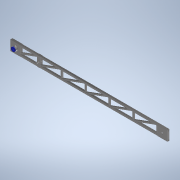
# Autodesk Inventor part: ms truss - 2
Saved by Autodesk Inventor 2020 (Build 240168000, 168)
## iProperties
Created: 2020-07-25
Part Number: ms truss - 2
Material: Steel, Mild
Document SubType Name: Modeling
Designer: Vikki
Mass: 14529.5 g
Surface Area: 14203.7 cm^2
Volume: 1850.9 cm^3
Density: 7.85 g/cm^3
Appearance: Semi-Polished
Author: Vikki
Autodesk Inventor part; units mm, degrees
ref_plane "YZ Plane" through (0, 0, 0) normal (1, 0, 0) x (0, 1, 0)
ref_plane "XZ Plane" through (0, 0, 0) normal (0, 1, 0) x (-1, 0, 0)
ref_plane "XY Plane" through (0, 0, 0) normal (0, 0, 1) x (1, 0, 0)
sketch "Sketch1" plane through (0, 0, 0) normal (1, 0, 0) x (0, 1, 0)
  line L0 (-12.7, 12.7) -> (12.7, 12.7)
  line L1 (12.7, 12.7) -> (12.7, -12.7)
  line L2 (12.7, -12.7) -> (-12.7, -12.7)
  line L3 (-12.7, -12.7) -> (-12.7, 12.7)
  line L4 (-12.7, 12.7) -> (12.7, -12.7) construction
  line L5 (12.7, 12.7) -> (-12.7, -12.7) construction
  line L6 (11.1, 11.1) -> (-11.1, 11.1)
  line L7 (-11.1, 11.1) -> (-11.1, -11.1)
  line L8 (-11.1, -11.1) -> (11.1, -11.1)
  line L9 (11.1, -11.1) -> (11.1, 11.1)
  line L10 (114.3, -11.1) -> (136.5, -11.1)
  line L11 (136.5, -11.1) -> (136.5, 11.1)
  line L12 (136.5, 11.1) -> (114.3, 11.1)
  line L13 (114.3, 11.1) -> (114.3, -11.1)
  line L14 (114.3, -11.1) -> (136.5, 11.1) construction
  line L15 (136.5, -11.1) -> (114.3, 11.1) construction
  line L16 (112.7, -12.7) -> (138.1, -12.7)
  line L17 (138.1, -12.7) -> (138.1, 12.7)
  line L18 (138.1, 12.7) -> (112.7, 12.7)
  line L19 (112.7, 12.7) -> (112.7, -12.7)
  line L20 (112.7, -12.7) -> (138.1, 12.7) construction
  line L21 (138.1, -12.7) -> (112.7, 12.7) construction
  point P0 (0, 0)
  point P1 (125.4, 0)
  point P2 (0, 0)
  point P3 (125.4, 0)
  dimension "d0" = 25.4
  dimension "d1" = 25.4
  dimension "d2" = 1.6
  dimension "d5" = 125.4
  constraints: 44 end point, 8 midpoint, 8 parallel, 4 equal length, 4 perpendicular, 3 horizontal, 1 horizontal alignment, 3 other
  measures "d0" distance of L1.end L2.end
  measures "d1" distance of L0.end L1.end
  measures "d2" distance between parallel lines of L0 L6
  measures "d5" distance of point (0, 0) point (125.4, 0)
extrude "Extrusion1" add sketch "Sketch1" along normal blind 2000
sketch "Sketch2" plane through (0, 12.7, 12.7) normal (0, 1, 0) x (1, 0, 0)
  line L0 (0, 25.4) -> (2000, 25.4) projected
  line L1 (0, 0) -> (25.4, 0)
  line L2 (25.4, 0) -> (25.4, 25.4)
  line L3 (25.4, 25.4) -> (0, 25.4)
  line L4 (0, 25.4) -> (0, 0)
  line L5 (2, 2) -> (23.4, 2)
  line L6 (23.4, 2) -> (23.4, 23.4)
  line L7 (23.4, 23.4) -> (2, 23.4)
  line L8 (2, 23.4) -> (2, 2)
  line L9 (2000, 0) -> (1974.6, 0)
  line L10 (1974.6, 0) -> (1974.6, 25.4)
  line L11 (1974.6, 25.4) -> (2000, 25.4)
  line L12 (2000, 25.4) -> (2000, 0)
  line L13 (1976.2, 1.6) -> (1998.4, 1.6)
  line L14 (1998.4, 1.6) -> (1998.4, 23.8)
  line L15 (1998.4, 23.8) -> (1976.2, 23.8)
  line L16 (1976.2, 23.8) -> (1976.2, 1.6)
  point P0 (0, 12.7)
  dimension "d6" = 25.4
  dimension "d7" = 2
  dimension "d8" = 25.4
  dimension "d9" = 1.6
  constraints: 32 end point, 8 parallel, 4 perpendicular, 2 horizontal, 2 point on line, 6 other
  measures "d6" distance of L1.start L1.end
  measures "d7" distance between parallel lines of L4 L8
  measures "d8" distance of L9.start L9.end
  measures "d9" distance between parallel lines of L13 L9
extrude "Extrusion2" add sketch "Sketch2" along normal up to surface (100 mm away)
sketch "Sketch3" plane through (25.4, 12.7, -12.7) normal (0, 1, 0) x (1, 0, 0)
  line L0 (90.2984, -21.425) -> (34.6, -21.425)
  line L1 (34.6, -21.425) -> (34.6, -2.375)
  line L2 (34.6, -2.375) -> (90.2984, -2.375)
  line L3 (90.2984, -2.375) -> (90.2984, -21.425)
  line L4 (-25.4, -23.8) -> (1974.6, -23.8) projected
  line L5 (-25.4, -23.8) -> (-25.4, -1.6) projected
  line L6 (89.0984, -20.225) -> (35.8, -20.225)
  line L7 (35.8, -20.225) -> (35.8, -3.575)
  line L8 (35.8, -3.575) -> (89.0984, -3.575)
  line L9 (89.0984, -3.575) -> (89.0984, -20.225)
  point P0 (-25.4, -12.7)
  point P1 (71.2484, -11.9)
  dimension "d12" = 19.05
  dimension "d13" = 55.6984
  dimension "d14" = 2.375
  dimension "d15" = 60
  dimension "d16" = 1.2
  dimension "d17" = 19.05
  dimension "d18" = 9.525
  constraints: 16 end point, 4 parallel, 2 perpendicular, 1 horizontal, 3 other
  measures "d12" distance of L0.end L1.end
  measures "d13" distance of L0.start L0.end
  measures "d14" distance between parallel lines of L0 L4
  measures "d15" distance between parallel lines of L1 L5
  measures "d16" distance between parallel lines of L3 L9
  measures "d17" distance from line of L3 point (71.248, -11.9)
  measures "d18" distance from line of L0 point (71.248, -11.9)
sketch "Sketch5" plane through (25.4, 112.7, 12.7) normal (0, -1, 0) x (1, 0, 0)
  point P0 (-25.4, -12.7)
  point P1 (71.2484, -13.5)
  point P2 (345.9961, -13.5)
  dimension "d19" = 274.7477
  constraints: 1 horizontal alignment
  measures "d19" distance of point (345.996, -13.5) point (71.248, -13.5)
sketch3d "3D Sketch1"
  line L0 (96.6484, 12.7, -0.8) -> (371.3961, 112.7, -0.8)
sweep "Sweep1" add profiles "Sketch3" path "3D Sketch1"
sketch "Sketch13" plane through (2000, -12.7, 12.7) normal (0, 0, 1) x (1, 0, 0)
  line L0 (0, 0) -> (-150, 0)
  line L1 (-150, 0) -> (-150, 150.8)
  line L2 (-150, 150.8) -> (0, 150.8)
  line L3 (0, 150.8) -> (0, 0)
  line L4 (-2000, 150.8) -> (0, 150.8) projected
  point P0 (-2000, 12.7)
  dimension "d60" = 150
  dimension "d133" = 0
  constraints: 8 end point, 2 parallel, 1 horizontal, 1 perpendicular
  measures "d60" distance of L1.end L2.end
  measures "d133" distance between parallel lines of L2 L4
sketch "Sketch17" plane through (25.4, 112.7, 12.7) normal (0, -1, 0) x (1, 0, 0)
  line L0 (370.0461, -3.975) -> (389.0961, -3.975)
  line L1 (389.0961, -3.975) -> (389.0961, -23.025)
  line L2 (389.0961, -23.025) -> (370.0461, -23.025)
  line L3 (370.0461, -23.025) -> (370.0461, -3.975)
  line L4 (309.3477, -3.975) -> (365.0461, -3.975) projected
  line L5 (365.0461, -23.025) -> (309.3477, -23.025) projected
  line L6 (365.0461, -3.975) -> (365.0461, -23.025) projected
  line L7 (371.0711, -22) -> (388.0711, -22)
  line L8 (388.0711, -22) -> (388.0711, -5)
  line L9 (388.0711, -5) -> (371.0711, -5)
  line L10 (371.0711, -5) -> (371.0711, -22)
  point P0 (-25.4, -12.7)
  dimension "d73" = 0
  dimension "d74" = 0
  dimension "d75" = 5
  dimension "d76" = 1.025
  constraints: 16 end point, 4 parallel, 3 perpendicular, 1 horizontal, 3 other
  measures "d73" distance between parallel lines of L0 L4
  measures "d74" distance between parallel lines of L5 L2
  measures "d75" distance between parallel lines of L6 L3
  measures "d76" distance between parallel lines of L2 L7
extrude "Extrusion14" add sketch "Sketch17" along normal up to surface (100 mm away)
pattern_linear "Rectangular Pattern3" count 5 spacing 357 along (1, 0, 0) of "Sweep1", "Extrusion14"
sketch "Sketch18" plane through (0, 0, 0) normal (-1, 0, 0) x (0, 0, 1)
  line L0 (-11.1, 136.5) -> (-11.1, 114.3) projected
  line L1 (11.1, 136.5) -> (-11.1, 136.5) projected
  line L2 (11.1, 114.3) -> (11.1, 136.5) projected
  line L3 (-11.1, 114.3) -> (11.1, 114.3) projected
  line L4 (12.7, 138.1) -> (12.7, -12.7) projected
  line L5 (-12.7, 138.1) -> (12.7, 138.1) projected
  line L6 (-12.7, -12.7) -> (-12.7, 138.1) projected
  line L7 (12.7, -12.7) -> (-12.7, -12.7) projected
  line L8 (-11.1, -11.1) -> (11.1, -11.1) projected
  line L9 (-11.1, 11.1) -> (-11.1, -11.1) projected
  line L10 (11.1, 11.1) -> (-11.1, 11.1) projected
  line L11 (11.1, -11.1) -> (11.1, 11.1) projected
  line L12 (-12.7, -12.7) -> (-12.7, 138.1) projected
  line L13 (-12.7, 112.7) -> (12.7, 112.7)
  line L14 (12.7, 138.1) -> (12.7, -12.7) projected
  line L15 (-12.7, 12.7) -> (12.7, 12.7)
  point P0 (0, 0)
  dimension "d82" = 1.6
  dimension "d83" = 1.6
  constraints: 4 end point, 4 point on line, 2 perpendicular
  measures "d82" distance between parallel lines of L13 L3
  measures "d83" distance between parallel lines of L10 L15
extrude "Extrusion15" add sketch "Sketch18" along normal blind 350 contours L4 L13 L6 L5 | L4 L7 L6 L15
sketch "Sketch20" plane through (25.4, 12.7, -12.7) normal (0, 0, -1) x (-1, 0, 0)
  line L0 (0, 0) -> (0, 100) projected
  line L1 (25.4, 0) -> (25.4, 100) projected
  line L2 (0, 100) -> (25.4, 100)
  line L3 (25.4, 100) -> (25.4, 0)
  line L4 (25.4, 0) -> (0, 0)
  line L5 (0, 0) -> (0, 100)
  point P0 (25.4, -12.7)
  point P1 (25.4, 100)
  constraints: 8 end point, 2 parallel, 1 horizontal, 1 perpendicular
extrude "Extrusion16" cut sketch "Sketch20" against normal blind 350
ref_plane "Work Plane5" through (1850, -12.7, -12.7) normal (0, 0, -1) x (-1, 0, 0)
sketch "Sketch22" plane through (1850, -12.7, -12.7) normal (0, 0, -1) x (-1, 0, 0)
  circle A0 centre (2125, 75.4) radius 15 projected
  line L0 (2200, 150.8) -> (0, 150.8) projected
  line L1 (2200, 1.6) -> (2050, 1.6)
  line L2 (2050, 1.6) -> (2050, 150.8)
  line L3 (2050, 150.8) -> (2200, 150.8)
  line L4 (2200, 150.8) -> (2200, 1.6)
  point P0 (1850, 12.7)
  point P1 (0, 150.8)
  dimension "d96" = 150
  constraints: 8 end point, 2 parallel, 1 horizontal, 1 perpendicular, 1 point on line
  measures "d96" distance of L1.start L1.end
extrude "Extrusion18" add sketch "Sketch22" along normal blind 4
sketch "Sketch23" plane through (-350, -12.7, 12.7) normal (0, 0, 1) x (1, 0, 0)
  line L0 (150, 1.6) -> (0, 1.6) projected
  line L1 (0, 1.6) -> (0, 150.8) projected
  line L2 (0, 150.8) -> (150, 150.8) projected
  line L3 (150, 150.8) -> (150, 1.6) projected
  circle A0 centre (75, 75.4) radius 15 projected
  point P0 (350, 12.7)
extrude "Extrusion19" add sketch "Sketch23" along normal blind 4
sketch "Sketch24" plane through (-350, -12.7, 16.7) normal (0, 0, 1) x (1, 0, 0)
  line L0 (150, 150.8) -> (0, 150.8) projected
  line L1 (0, 150.8) -> (0, 1.6) projected
  line L2 (0, 1.6) -> (150, 1.6) projected
  line L3 (150, 1.6) -> (150, 150.8) projected
  circle A0 centre (75, 75.4) radius 15 projected
  circle A1 centre (75, 75.4) radius 35
  circle A2 centre (75, 75.4) radius 31
  point P0 (350, 12.7)
  dimension "d101" = 70
  dimension "d104" = 62
  constraints: 2 centre point, 2 coincident
  measures "d101" diameter of A1
  measures "d104" diameter of A2
extrude "Extrusion20" add sketch "Sketch24" along normal blind 25 contours A1
sketch "Sketch26" plane through (1850, -12.7, -16.7) normal (0, 0, -1) x (-1, 0, 0)
  circle A0 centre (2125, 75.4) radius 35 projected
  circle A1 centre (2125, 75.4) radius 31 projected
  point P0 (1850, 12.7)
extrude "Extrusion21" add sketch "Sketch26" along normal blind 25
fillet "Fillet1" radius 8 1 edges at (-310, 62.7, 16.7)
fillet "Fillet3" radius 5 2 edges at (-200, 125.4, 12.7) (-200, 0.8, 12.7)
sketch "Sketch28" plane through (-350, -12.7, 12.7) normal (0, 0, 1) x (1, 0, 0)
  circle A0 centre (425, 75.4) radius 12.5
  circle A1 centre (75, 75.4) radius 15 projected
  point P0 (350, 12.7)
  dimension "d110" = 350
  dimension "d111" = 25
  dimension "d126" = 0
  constraints: 1 centre point
  measures "d110" distance of A0.centre A1.centre
  measures "d111" diameter of A0
  measures "d126" vertical distance of A1.centre A0.centre
extrude "Extrusion22" add sketch "Sketch28" along normal blind 40 and the other way blind 65.4 contours A0
sketch "Sketch29" plane through (75, 62.7, 52.7) normal (0, 0, 1) x (1, 0, 0)
  circle A0 centre (0, 0) radius 12.5 projected
  circle A1 centre (0, 0) radius 10
  point P0 (-75, -62.7)
  dimension "d116" = 20
  constraints: 1 centre point, 1 coincident
  measures "d116" diameter of A1
extrude "Extrusion23" cut sketch "Sketch29" against normal blind 30
sketch "Sketch30" plane through (75, 62.7, -52.7) normal (0, 0, -1) x (-1, 0, 0)
  circle A0 centre (0, 0) radius 12.5 projected
  circle A1 centre (0, 0) radius 10
  point P0 (75, -62.7)
  dimension "d119" = 20
  constraints: 1 centre point, 1 coincident
  measures "d119" diameter of A1
extrude "Extrusion24" cut sketch "Sketch30" against normal blind 30
sketch "Sketch33" plane through (-195.101, 112.7, 12.7) normal (0, 0, 1) x (1, 0, 0)
  line L0 (-4.899, 25.4) -> (2195.101, 25.4) projected
  line L1 (245.101, 25.4) -> (295.101, 25.4)
  line L2 (295.101, 25.4) -> (295.101, -125.4)
  line L3 (295.101, -125.4) -> (245.101, -125.4)
  line L4 (245.101, -125.4) -> (245.101, 25.4)
  line L5 (-154.899, -125.4) -> (2195.101, -125.4) projected
  circle A0 centre (270.101, -50) radius 10 projected
  circle A1 centre (270.101, -50) radius 12.5 projected
  point P0 (195.101, -112.7)
  point P1 (0, 25.4)
  point P2 (2045.101, 25.4)
  point P3 (2045.101, -125.4)
  point P4 (295.101, 25.4)
  point P5 (-154.899, 25.4)
  dimension "d127" = 50
  dimension "d128" = 25
  constraints: 8 end point, 2 parallel, 1 collinear, 1 horizontal, 1 perpendicular, 1 point on line
  measures "d127" distance of L2.end L3.end
  measures "d128" distance from line of L4 A1.centre
extrude "Extrusion26" add sketch "Sketch33" along normal blind 4 contours L0 L2 L3 L4
ref_plane "Work Plane6" through (1850, -12.7, -12.7) normal (0, 0, -1) x (-1, 0, 0)
sketch "Sketch34" plane through (1850, -12.7, -12.7) normal (0, 0, -1) x (-1, 0, 0)
  line L0 (1800, 150.8) -> (1800, 0) projected
  line L1 (1800, 0) -> (1750, 0) projected
  line L2 (1750, 0) -> (1750, 150.8) projected
  line L3 (1750, 150.8) -> (1800, 150.8) projected
  circle A0 centre (1775, 75.4) radius 12.5 projected
  point P0 (1850, 12.7)
extrude "Extrusion27" add sketch "Sketch34" along normal blind 4
pattern_linear "Rectangular Pattern5" count 2 spacing 325 along (-1, 0, 0) of "Sweep1"
ref_plane "Work Plane7" through (75, 62.7, 42.7) normal (0, 0, 1) x (1, 0, 0)
sketch "Sketch35" plane through (75, 62.7, 42.7) normal (0, 0, 1) x (1, 0, 0)
  circle A0 centre (0, 0) radius 10 projected
  circle A1 centre (0, 0) radius 9
  point P0 (-75, -62.7)
  dimension "d138" = 18
  constraints: 1 centre point, 1 coincident
  measures "d138" diameter of A1
extrude "Extrusion28" cut sketch "Sketch35" along normal blind 1 and the other way blind 2
ref_plane "Work Plane8" through (75, 62.7, 0) normal (0, 0, 1) x (1, 0, 0)
mirror "Mirror3" about plane through (75, 62.7, 0) normal (0, 0, 1) of "Extrusion28"
sketch "Sketch36" plane through (2000, -12.7, 12.7) normal (0, 0, 1) x (1, 0, 0)
  line L0 (-145, 144.2) -> (-5, 144.2)
  line L1 (-5, 144.2) -> (-5, 5)
  line L2 (-5, 5) -> (-145, 5)
  line L3 (-145, 5) -> (-145, 144.2)
  line L4 (-2350, 149.2) -> (0, 149.2) projected
  line L5 (-1900, 0) -> (0, 0) projected
  line L6 (0, 150.8) -> (0, 0) projected
  circle A0 centre (-75, 75.4) radius 12.75
  circle A1 centre (-2275, 75.4) radius 15 projected
  point P0 (-2000, 12.7)
  dimension "d141" = 5
  dimension "d142" = 5
  dimension "d143" = 5
  dimension "d144" = 25.5
  dimension "d145" = 140
  dimension "d146" = 2200
  constraints: 8 end point, 2 parallel, 1 centre point, 1 horizontal, 1 horizontal alignment, 1 perpendicular
  measures "d141" distance between parallel lines of L4 L0
  measures "d142" distance between parallel lines of L5 L2
  measures "d143" distance between parallel lines of L6 L1
  measures "d144" diameter of A0
  measures "d145" distance of L0.start L0.end
  measures "d146" distance of A1.centre A0.centre
extrude "Extrusion29" add sketch "Sketch36" along normal blind 4 contours L0 L1 L2 L3
sketch "Sketch37" plane through (2000, -12.7, -12.7) normal (0, 0, -1) x (-1, 0, 0)
  line L0 (145, 144.2) -> (145, 5) projected
  line L1 (145, 5) -> (5, 5) projected
  line L2 (5, 5) -> (5, 144.2) projected
  line L3 (5, 144.2) -> (145, 144.2) projected
  circle A0 centre (75, 75.4) radius 12.75 projected
  line L4 (145, 5) -> (5, 5) projected
  line L5 (45, 5) -> (45, 144.2)
  line L6 (105, 5) -> (105, 144.2)
  line L7 (5, 144.2) -> (145, 144.2) projected
  point P0 (2000, 12.7)
  point P1 (105, 5)
  point P2 (105, 144.2)
  point P3 (45, 5)
  dimension "d149" = 60
  dimension "d150" = 40
  constraints: 4 end point, 4 point on line, 2 perpendicular
  measures "d149" distance between parallel lines of L6 L5
  measures "d150" distance between parallel lines of L2 L5
extrude "Extrusion30" add sketch "Sketch37" along normal blind 4 contours L6 L1 L5 L3
sketch "Sketch38" plane through (2000, -12.7, -16.7) normal (0, 0, -1) x (-1, 0, 0)
  circle A0 centre (75, 75.4) radius 12.75 projected
  circle A1 centre (75, 75.4) radius 25
  point P0 (2000, 12.7)
  dimension "d156" = 50
  constraints: 1 centre point, 1 coincident
  measures "d156" diameter of A1
extrude "Extrusion31" cut sketch "Sketch38" against normal blind 1
sketch "Sketch41" plane through (2000, -12.7, 16.7) normal (0, 0, 1) x (1, 0, 0)
  line L0 (-145, 5) -> (-5, 5) projected
  line L1 (-5, 5) -> (-5, 144.2) projected
  line L2 (-5, 144.2) -> (-145, 144.2) projected
  line L3 (-145, 144.2) -> (-145, 5) projected
  circle A0 centre (-75, 75.4) radius 12.75 projected
  point P0 (-2000, 12.7)
extrude "Extrusion33" add sketch "Sketch41" along normal blind 4
sketch "Sketch48" plane through (-275, 62.7, 41.7) normal (0, 0, 1) x (1, 0, 0)
  circle A0 centre (0, 0) radius 31 projected
  circle A1 centre (0, 0) radius 15 projected
  point P0 (275, -62.7)
extrude "Extrusion39" add sketch "Sketch48" along normal mid plane 20
mirror "Mirror4" about plane through (75, 62.7, 0) normal (0, 0, 1) of "Extrusion39"
equation "\"d6\" = d0"
equation "\"d8\" = d0"
body "Solid1"
